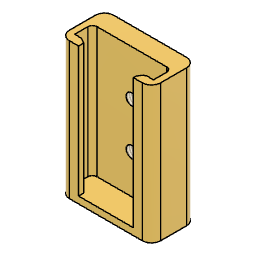
bracket_bluetooth v7 (Autodesk Fusion 360 design; units mm, degrees)
Autodesk Fusion 360 part; units mm, degrees
note: some values were not read from the file. Set by a fixed rule: which face or edge a step refers to.
sketch "Sketch1" plane through (0, 0, 0) normal (0, 0, 1) x (1, 0, 0)
  line L0 (10, 15) -> (-10, 15)
  line L1 (-10, 15) -> (-10, -15)
  line L2 (-10, -15) -> (10, -15)
  line L3 (10, -15) -> (10, 15)
  line L4 (10, 15) -> (-10, -15) construction
  line L5 (-10, 15) -> (10, -15) construction
  line L6 (0, -15) -> (0, 15) construction
  circle A0 centre (0, 5) radius 1.5
  line L7 (0, 0) -> (10, 0) construction
  circle A1 centre (0, -5) radius 1.5
  dimension "d1" = 20
  dimension "d2" = 30
  dimension "d3" = 3
  dimension "d4" = 5
  constraint horizontal L0
  constraint perpendicular L0 L1
  constraint parallel L0 L2
  constraint parallel L1 L3
  constraint coincident L4 L7.start
  constraint coincident L5 L7.start
  constraint coincident L7.start origin
  constraint midpoint L2 L6.start
  constraint midpoint L0 L6.end
  constraint coincident L6 A0.centre
  constraint midpoint L3 L7.end
  constraint symmetric A0 L7 A1
  measures "d1" distance of L1.end L2.end
  measures "d2" distance of L0.end L1.end
  measures "d3" diameter of A0
  measures "d4" distance of L7.start A0.centre
extrude "Extrude1" add sketch "Sketch1" against normal blind 3
sketch "Sketch2" plane through (0, 0, 0) normal (0, 1, 0) x (1, 0, 0)
  line L0 (10, 0) -> (-10, 0)
  line L1 (-10, 0) -> (-10, 3)
  line L2 (-10, 3) -> (10, 3)
  line L3 (10, 3) -> (10, 0)
  line L4 (-10, 0) -> (-6, 0)
  line L5 (-6, 0) -> (-6, -5.7)
  line L6 (-6, -5.7) -> (-10, -5.7)
  line L7 (-10, -5.7) -> (-10, 0)
  line L8 (0, 0) -> (0, 3) construction
  line L9 (10, -5.7) -> (10, 0)
  line L10 (10, 0) -> (6, 0)
  line L11 (6, 0) -> (6, -5.7)
  line L12 (6, -5.7) -> (10, -5.7)
  line L13 (-6, -3.7) -> (-10, -3.7)
  line L14 (6, -3.7) -> (10, -3.7)
  line L15 (10, 0) -> (8.45, 0)
  line L16 (8.45, 0) -> (8.45, -5.7)
  line L17 (8.45, -5.7) -> (10, -5.7)
  line L18 (10, -5.7) -> (10, 0)
  line L19 (-10, -5.7) -> (-10, 0)
  line L20 (-10, 0) -> (-8.45, 0)
  line L21 (-8.45, 0) -> (-8.45, -5.7)
  line L22 (-8.45, -5.7) -> (-10, -5.7)
  dimension "d9" = 3.7
  dimension "d10" = 2
  dimension "d11" = 16.9
  constraint horizontal L4
  constraint vertical L5
  constraint horizontal L6
  constraint vertical L7
  constraint coincident L0.end L1.start
  constraint coincident L8.start origin
  constraint midpoint L2 L8.end
  constraint symmetric L0.end L8 L0.start
  constraint symmetric L4.end L8 L10.end
  constraint symmetric L5.end L8 L11.end
  constraint symmetric L6.end L8 L9.start
  constraint coincident L5 L13.start
  constraint coincident L7 L13.end
  constraint perpendicular L7 L13
  constraint symmetric L8 L13.start L14.start
  constraint symmetric L8 L13.end L14.end
  constraint horizontal L15
  constraint vertical L16
  constraint horizontal L17
  constraint vertical L18
  constraint coincident L12 L16.end
  constraint coincident L0.start L3.end
  constraint symmetric L8 L0.start L0.end
  constraint symmetric L8 L15.end L20.end
  constraint symmetric L8 L16.end L21.end
  constraint symmetric L8 L9.start L6.end
  measures "d9" distance of L4 L13
  measures "d10" distance of L6 L13
  measures "d11" distance of L16 L21
extrude "Extrude2" add sketch "Sketch2" along normal mid plane 30 contours L0 L9 L10 L14 L15 L16 L18 | L9 L12 L14 L16 L17 L18 | L11 L12 L14 L16 | L0 L4 L7 L13 L19 L20 L21 | L5 L6 L13 L21 | L6 L7 L13 L19 L21 L22
thread "Thread1" "ISO Metric profile 3.0 M3x0.5 6H" major diameter 3.086 minor diameter 2.529 pitch 0.5 angle 60 resizes the face on face at (1.4981, -5.0748, -2) on face at (1.4981, 4.9252, -2)
chamfer "Chamfer1" distance 1.5 angle 30 2 edges at (-6, 0, 3.7) (6, 0, 3.7) measured on face at (-6.8167, -5, 3.7) measured on face at (6, 5, 5.0333)
fillet "Fillet1" radius 1 2 edges at (-8.45, 0, 0) (8.45, 0, 0)
sketch "Sketch3" plane through (0, -15, 0) normal (0, -1, 0) x (1, 0, 0)
  line L0 (6, 5.2) -> (6.866, 3.7)
  line L1 (6.866, 3.7) -> (8.45, 3.7)
  line L2 (8.45, 3.7) -> (8.45, 1)
  arc A0 (7.45, 0) -> (8.45, 1) centre (7.45, 1) ccw
  line L3 (7.45, 0) -> (-7.45, 0)
  arc A1 (-8.45, 1) -> (-7.45, 0) centre (-7.45, 1) ccw
  line L4 (-8.45, 1) -> (-8.45, 3.7)
  line L5 (-8.45, 3.7) -> (-7.5, 3.7)
  line L6 (-7.5, 3.7) -> (-6, 4.566)
  line L7 (-6, 4.566) -> (-6, 5.7)
  line L8 (-6, 5.7) -> (-10, 5.7)
  line L9 (-10, 5.7) -> (-10, -3)
  line L10 (-10, -3) -> (10, -3)
  line L11 (10, -3) -> (10, 5.7)
  line L12 (10, 5.7) -> (6, 5.7)
  line L13 (6, 5.7) -> (6, 5.2)
  line L14 (-6, 5.7) -> (6, 5.7)
  constraint coincident L7.end L8.start
  constraint coincident L12.end L13.start
extrude "Extrude3" add sketch "Sketch3" against normal blind 1.5 contours L0 L1 L2 A0 L3 A1 L4 L5 L6 L7 L13 L14
fillet "Fillet2" radius 2 4 edges at (10, 0, 5.7) (10, 0, -3) (-10, 0, -3) (-10, 0, 5.7)
fillet "Fillet3" radius 1 2 edges at (6.866, 0.75, 3.7) (-7.5, 0.75, 3.7)
move_face "OffsetFaces1" offset -0.2 2 faces at (-8.45, 5.5, 2.8) (8.45, 5.5, 2.8)
move_face "OffsetFaces2" offset -0.2 2 faces at (7.8456, -4, 3.7) (-8.062, -4, 3.7)
move_face "OffsetFaces3" offset 1 1 faces at (0.0315, -12.087, -3)
